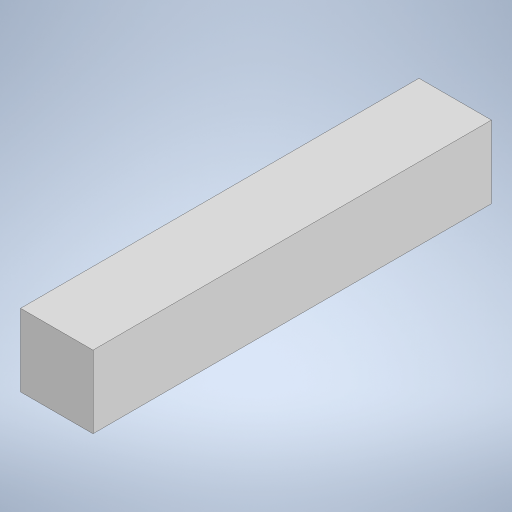
# Autodesk Inventor part: camera-back-support
Saved by Autodesk Inventor 2023 (Build 270158000, 158)
## iProperties
Created: 2024-04-10
Part Number: camera-back-support
Material: Genérico
Document SubType Name: Modeling
Designer: inigo
Density: 1 g/cm^3
Appearance: Valor por defecto
Author: inigo
Autodesk Inventor part; units mm, degrees
ref_plane "YZ Plane" through (0, 0, 0) normal (1, 0, 0) x (0, 1, 0)
ref_plane "XZ Plane" through (0, 0, 0) normal (0, 1, 0) x (-1, 0, 0)
ref_plane "XY Plane" through (0, 0, 0) normal (0, 0, 1) x (1, 0, 0)
sketch "Boceto1" plane through (0, 0, 0) normal (0, 1, 0) x (-1, 0, 0)
  line L0 (1.5, 8.25) -> (-1.5, 8.25)
  line L1 (-1.5, 8.25) -> (-1.5, -8.25)
  line L2 (-1.5, -8.25) -> (1.5, -8.25)
  line L3 (1.5, -8.25) -> (1.5, 8.25)
  line L4 (1.5, 8.25) -> (-1.5, -8.25) construction
  line L5 (-1.5, 8.25) -> (1.5, -8.25) construction
  point P0 (0, 0)
  dimension "d0" = 3
  dimension "d1" = 16.5
  constraints: 12 end point, 2 midpoint, 2 parallel, 1 horizontal, 1 perpendicular
  measures "d0" distance of L2.end L1.end
  measures "d1" distance of L1.end L0.end
extrude "Extrusión1" add sketch "Boceto1" along normal blind 3
